NoOffset v6 (Autodesk Fusion 360 design; units mm, degrees)
Autodesk Fusion 360 part; units mm, degrees
sketch "Sketch1" plane through (0, 0, 0) normal (0, 1, 0) x (1, 0, 0)
  circle A0 centre (0, 0) radius 32.5
  circle A1 centre (0, 0) radius 28.5
  dimension "d1" = 65
  dimension "d2" = 57
  constraint coincident A0.centre A1.centre
  measures "d1" diameter of A0
  measures "d2" diameter of A1
extrude "Extrude1" add sketch "Sketch1" along normal blind 10 makes body 1
sketch "Sketch2" plane through (0, 10, 0) normal (0, 1, 0) x (-1, 0, 0)
  circle A0 centre (0, 0) radius 28.5
  circle A1 centre (0, 0) radius 32.5
  circle A2 centre (0, 0) radius 28.5
  circle A3 centre (0, 0) radius 27.5
  dimension "d5" = -1
extrude "Extrude2" add sketch "Sketch2" along normal blind 30 separate body contours A0 A2 makes body 2
chamfer "Chamfer1" distance 0.5 angle 45 1 edges at (26.5713, 40, -10.306) on bodies 2
ref_plane "WorkPlane1" through (28.5, 15.6684, 0) normal (1, 0, 0) x (0, 0, 1)
sketch "Sketch3" plane through (28.5, 15.6684, 0) normal (1, 0, 0) x (0, 0, -1)
  line L0 (28.5, -5.6684) -> (-28.5, -5.6684) construction
  line L1 (28.5, 23.8316) -> (-28.5, 23.8316) construction
  line L2 (0, 23.8316) -> (0, -5.6684)
  line L3 (0, 9.0816) -> (10.0781, 9.0816) construction
  line L4 (10.0781, 9.0816) -> (10.0781, 16.0492) construction
  line L5 (10.0781, 16.0492) -> (0, 16.0492) construction
  line L6 (0, 16.0492) -> (0, 9.0816) construction
  dimension "d10" = 10
  text T0 "No" font "Arial" height 10 align centre middle in box 10.0781 x 6.9676 at (0, 9.0816) x (1, 0) y (0, 1) spacing 1
  constraint midpoint L1 L2.start
  constraint midpoint L0 L2.end
  constraint midpoint L2
emboss "Emboss1" depth -2 profiles "Sketch3" section 1 text T0 onto face at (-28.4646, 29.6667, -1.4206) on bodies 2 bodies 2 makes body 3 at (26.9913, 28.6901, -9.1499)
delete_body "RemoveBody1" bodies 3
move_face "OffsetFaces1" offset 1 1 faces at (-27.9582, 10, -2.7821) on bodies 2
combine "Combine1" operation add target body 2 tool bodies 1
